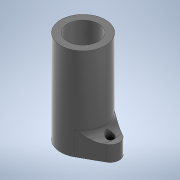
# Autodesk Inventor part: Antenna_cover_01
Saved by Autodesk Inventor 2020 (Build 240168000, 168)
## iProperties
Created: 2021-08-14
Part Number: Antenna_cover_01
Material: アセタール樹脂、黒
Document SubType Name: Modeling
Designer: Masato
Density: 1.425 g/cm^3
Appearance: 滑らか - 黒
Author: Masato
Autodesk Inventor part; units mm, degrees
ref_plane "YZ Plane" through (0, 0, 0) normal (1, 0, 0) x (0, 1, 0)
ref_plane "XZ Plane" through (0, 0, 0) normal (0, 1, 0) x (-1, 0, 0)
ref_plane "XY Plane" through (0, 0, 0) normal (0, 0, 1) x (1, 0, 0)
sketch "スケッチ1" plane through (0, 0, 0) normal (0, 0, 1) x (1, 0, 0)
  circle A0 centre (0, 0) radius 5
  circle A1 centre (-8.75, 0) radius 1.25
  arc A2 (-10.2071, 2.6224) -> (-10.2071, -2.6224) centre (-8.75, 0) ccw
  line L0 (0, 0) -> (-11.75, 0) construction
  line L1 (0, 7.25) -> (0, -7.25) construction
  line L2 (-10.2071, 2.6224) -> (-3.5214, 6.3374)
  arc A3 (-3.5214, -6.3374) -> (-3.5214, 6.3374) centre (0, 0) ccw
  line L3 (-10.2071, -2.6224) -> (-3.5214, -6.3374)
  arc A4 (-3.5214, 6.3374) -> (-3.5214, -6.3374) centre (0, 0) ccw
  point P0 (-7.2323, -0.5066)
  point P1 (-7.2323, 0.5066)
  dimension "d0" = 10
  dimension "d2" = 2.5
  dimension "d3" = 6
  dimension "d4" = 8.75
  dimension "d6" = 7.25
  constraints: 9 point on circle, 8 end point, 5 centre point, 4 coincident, 4 tangent, 1 midpoint, 1 perpendicular, 1 point on line, 1 vertical
  measures "d0" diameter of A0
  measures "d2" diameter of A1
  measures "d3" diameter of A2
  measures "d4" distance of point (0, 0) A1.centre
  measures "d6" radius of A3
extrude "押し出し1" add sketch "スケッチ1" along normal blind 30 contours A3 A4
extrude "押し出し2" add sketch "スケッチ1" along normal blind 5 contours L2 A4 L3 A2
fillet "フィレット1" radius 2.7 1 edges at (-7.25, 0, 5)
